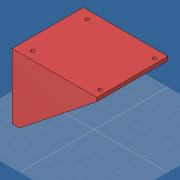
# Autodesk Inventor part: Sanftanlauf_Halter
Saved by Autodesk Inventor 2019 (Build 230136000, 136)
## iProperties
Created: 2020-08-07
Part Number: Sanftanlauf_Halter
Material: Generisch
Document SubType Name: Modeling
Designer: Stefan
Mass: 37.6604 g
Surface Area: 217.27 cm^2
Volume: 37.6604 cm^3
Density: 1 g/cm^3
Appearance: Glatt - Rot
Author: Stefan
Autodesk Inventor part; units mm, degrees
ref_plane "YZ Plane" through (0, 0, 0) normal (1, 0, 0) x (0, 1, 0)
ref_plane "XZ Plane" through (0, 0, 0) normal (0, 1, 0) x (-1, 0, 0)
ref_plane "XY Plane" through (0, 0, 0) normal (0, 0, 1) x (1, 0, 0)
sketch "Skizze1" plane through (0, 0, 0) normal (0, 1, 0) x (-1, 0, 0)
  line L0 (-31.5, -26) -> (31.5, -26)
  line L1 (31.5, -26) -> (31.5, 26)
  line L2 (31.5, 26) -> (-31.5, 26)
  line L3 (-31.5, 26) -> (-31.5, -26)
  line L4 (-31.5, -26) -> (31.5, 26) construction
  line L5 (31.5, -26) -> (-31.5, 26) construction
  circle A0 centre (27.5, 22.25) radius 1.5
  circle A1 centre (-27.5, 22.25) radius 1.5
  circle A2 centre (-27.5, -22.25) radius 1.5
  circle A3 centre (27.5, -22.25) radius 1.5
  line L6 (31.5, 0) -> (-31.5, 0) construction
  line L7 (0, 26) -> (0, -26) construction
  line L8 (31.5, -26) -> (31.5, 26)
  line L9 (31.5, 26) -> (37.5, 26)
  line L10 (37.5, 26) -> (37.5, -26)
  line L11 (37.5, -26) -> (31.5, -26)
  point P0 (0, 0)
  dimension "d0" = 63
  dimension "d1" = 52
  dimension "d4" = 3
  dimension "d9" = 44.5
  dimension "d10" = 55
  dimension "d11" = 6
  constraints: 24 end point, 6 midpoint, 4 centre point, 4 parallel, 3 equal radius, 2 horizontal alignment, 2 perpendicular, 2 symmetric about line, 2 vertical alignment, 1 horizontal, 1 vertical
  measures "d0" distance of L1.end L2.end
  measures "d1" distance of L0.end L1.end
  measures "d4" diameter of A0
  measures "d9" distance of A3.centre A0.centre
  measures "d10" distance of A1.centre A0.centre
  measures "d11" distance of L1.end L9.end
extrude "Extrusion1" add sketch "Skizze1" along normal blind 3
extrude "Extrusion2" add sketch "Skizze1" against normal blind 50 contours L1 L9 L10 L11
sketch "Skizze2" plane through (-31.5, -50, 26) normal (1, 0, 0) x (0, 0, -1)
  line L0 (52, 0) -> (0, 0) projected
  line L1 (26, 50) -> (26, 0) construction
  line L2 (7.5, 6.5) -> (44.5, 6.5)
  line L3 (44.5, 6.5) -> (44.5, 43.5)
  line L4 (44.5, 43.5) -> (7.5, 43.5)
  line L5 (7.5, 43.5) -> (7.5, 6.5)
  line L6 (7.5, 6.5) -> (44.5, 43.5) construction
  line L7 (44.5, 6.5) -> (7.5, 43.5) construction
  line L8 (42.9123, 3.75) -> (41.3246, 6.5)
  line L9 (41.3246, 6.5) -> (42.9123, 9.25)
  line L10 (42.9123, 9.25) -> (46.0877, 9.25)
  line L11 (46.0877, 9.25) -> (47.6754, 6.5)
  line L12 (47.6754, 6.5) -> (46.0877, 3.75)
  line L13 (46.0877, 3.75) -> (42.9123, 3.75)
  line L14 (5.9123, 3.75) -> (4.3246, 6.5)
  line L15 (4.3246, 6.5) -> (5.9123, 9.25)
  line L16 (5.9123, 9.25) -> (9.0877, 9.25)
  line L17 (9.0877, 9.25) -> (10.6754, 6.5)
  line L18 (10.6754, 6.5) -> (9.0877, 3.75)
  line L19 (9.0877, 3.75) -> (5.9123, 3.75)
  line L20 (41.3246, 43.5) -> (42.9123, 46.25)
  line L21 (42.9123, 46.25) -> (46.0877, 46.25)
  line L22 (46.0877, 46.25) -> (47.6754, 43.5)
  line L23 (47.6754, 43.5) -> (46.0877, 40.75)
  line L24 (46.0877, 40.75) -> (42.9123, 40.75)
  line L25 (42.9123, 40.75) -> (41.3246, 43.5)
  line L26 (4.3246, 43.5) -> (5.9123, 46.25)
  line L27 (5.9123, 46.25) -> (9.0877, 46.25)
  line L28 (9.0877, 46.25) -> (10.6754, 43.5)
  line L29 (10.6754, 43.5) -> (9.0877, 40.75)
  line L30 (9.0877, 40.75) -> (5.9123, 40.75)
  line L31 (5.9123, 40.75) -> (4.3246, 43.5)
  circle A0 centre (44.5, 6.5) radius 1.75
  circle A1 centre (7.5, 6.5) radius 1.75
  circle A2 centre (44.5, 43.5) radius 1.75
  circle A3 centre (7.5, 43.5) radius 1.75
  circle A4 centre (26, 25) radius 4
  point P0 (26, 25)
  dimension "d30" = 37
  dimension "d31" = 37
  dimension "d39" = 5.5
  dimension "d42" = 3.5
  dimension "d45" = 8
  constraints: 62 end point, 8 coincident, 6 midpoint, 5 centre point, 5 horizontal, 3 equal length, 3 equal radius, 2 parallel, 1 perpendicular, 52 other
  measures "d30" distance of L3.end L4.end
  measures "d31" distance of L4.end L2.start
  measures "d39" distance between parallel lines of L10 L13
  measures "d42" diameter of A0
  measures "d45" diameter of A4
extrude "Extrusion4" cut sketch "Skizze2" against normal through all contours L5 A1 L2 | L2 A1 L5 | A0 L3 L2 | L2 L3 A0 | A3 L4 L5 | L5 L4 A3 | A2 L4 L3 | L3 L4 A2 | A4
extrude "Extrusion3" cut sketch "Skizze2" against normal blind 3 contours L5 A1 L2 | L2 A1 L5 | A1 L5 L16 L17 L2 | L2 L18 L19 L14 L15 L16 L5 A1 | L9 L10 L3 A0 L2 | L2 A0 L3 L10 L11 L12 L13 L8 | L30 L31 L26 L27 L28 L4 A3 L5 | L5 A3 L4 L29 L30 | A0 L3 L2 | L2 L3 A0 | A3 L4 L5 | L5 L4 A3 | L24 L25 L4 A2 L3 | L3 A2 L4 L20 L21 L22 L23 L24 | A2 L4 L3 | L3 L4 A2
sketch "Skizze3" plane through (31.5, 3, -26) normal (0, 0, -1) x (-1, 0, 0)
  line L0 (0, -3) -> (63, -3) projected
  line L1 (63, -3) -> (63, -53) projected
  line L2 (69, -53) -> (63, -53) projected
  line L3 (69, -53) -> (69, 0) projected
  line L4 (0, 0) -> (69, 0) projected
  line L5 (0, -3) -> (0, 0) projected
  line L6 (63, -53) -> (0, -3)
  point P0 (31.5, -3)
  constraints: 2 end point
extrude "Extrusion5" add sketch "Skizze3" along normal blind 3
sketch "Skizze4" plane through (-37.5, 3, 26) normal (0, 0, 1) x (1, 0, 0)
  line L0 (6, -3) -> (69, -3) projected
  line L1 (69, -3) -> (69, 0) projected
  line L2 (0, 0) -> (69, 0) projected
  line L3 (0, -53) -> (0, 0) projected
  line L4 (6, -53) -> (0, -53) projected
  line L5 (6, -3) -> (6, -53) projected
  line L6 (6, -53) -> (69, -3)
  point P0 (37.5, -3)
  constraints: 2 end point
extrude "Extrusion6" add sketch "Skizze4" along normal blind 3
sketch "Skizze5" plane through (-37.5, -50, -29) normal (-1, 0, 0) x (0, 0, 1)
  circle A0 centre (29, 25) radius 4 projected
  circle A1 centre (29, 25) radius 7.5
  point P0 (29, 50)
  dimension "d51" = 15
  constraints: 1 centre point, 1 coincident
  measures "d51" diameter of A1
extrude "Extrusion7" cut sketch "Skizze5" against normal blind 3
equation "\"d31\" = d30"
